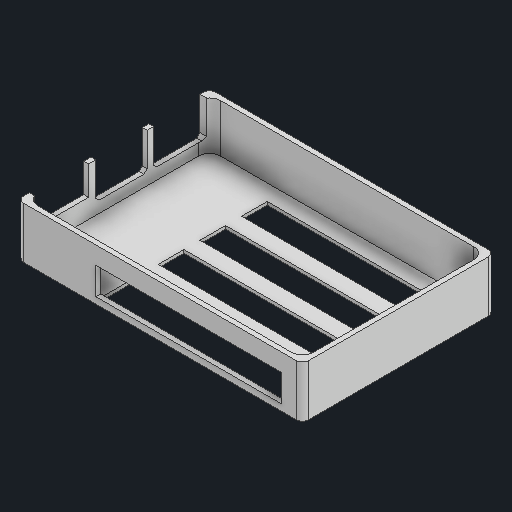
# Autodesk Inventor part: raspi_cover
Saved by Autodesk Inventor 2025 (Build 290162010, 162A)
## iProperties
Created: 2024-09-11
Part Number: raspi_cover
Material: Generic
Document SubType Name: Modeling
Designer: mihir
Density: 1 g/cm^3
Appearance: Default
Author: mihir
Autodesk Inventor part; units mm, degrees
ref_plane "YZ Plane" through (0, 0, 0) normal (1, 0, 0) x (0, 1, 0)
ref_plane "XZ Plane" through (0, 0, 0) normal (0, 1, 0) x (-1, 0, 0)
ref_plane "XY Plane" through (0, 0, 0) normal (0, 0, 1) x (1, 0, 0)
sketch "Sketch1" plane through (0, 0, 0) normal (0, 1, 0) x (-1, 0, 0)
  line L0 (2, 0) -> (87, 0)
  line L1 (89, -2) -> (89, -58)
  line L2 (87, -60) -> (2, -60)
  line L3 (0, -58) -> (0, -2)
  arc A0 (2, 0) -> (0, -2) centre (2, -2) ccw
  arc A1 (0, -58) -> (2, -60) centre (2, -58) ccw
  arc A2 (87, -60) -> (89, -58) centre (87, -58) ccw
  arc A3 (89, -2) -> (87, 0) centre (87, -2) ccw
  point P0 (0, 0)
  point P1 (89, -60)
  point P2 (0, -60)
  dimension "d0" = 60
  dimension "d1" = 89
  dimension "d2" = 2
  constraints: 8 end point, 8 point on circle, 8 tangent, 6 point on line, 4 centre point, 3 equal radius, 2 parallel, 1 horizontal, 1 perpendicular
  measures "d0" distance of point (0, -60) point (0, 0)
  measures "d1" distance of point (89, -60) point (0, -60)
  measures "d2" radius of A0
extrude "Extrusion1" add sketch "Sketch1" along normal blind 1
sketch "Sketch2" plane through (0, 1, 0) normal (0, 1, 0) x (1, 0, 0)
  line L0 (-87, 0) -> (-2, 0)
  line L1 (0, 2) -> (0, 58)
  line L2 (-2, 60) -> (-87, 60)
  line L3 (-89, 58) -> (-89, 2)
  line L4 (-89, 58) -> (-89, 2) projected
  line L5 (-87, 0) -> (-2, 0) projected
  line L6 (0, 2) -> (0, 58) projected
  line L7 (-2, 60) -> (-87, 60) projected
  arc A0 (-89, 2) -> (-87, 0) centre (-87, 2) ccw
  arc A1 (-87, 60) -> (-89, 58) centre (-87, 58) ccw
  arc A2 (0, 58) -> (-2, 60) centre (-2, 58) ccw
  arc A3 (-2, 0) -> (0, 2) centre (-2, 2) ccw
  line L8 (-84, 1.5) -> (-5, 1.5)
  line L9 (-1.5, 5) -> (-1.5, 55)
  line L10 (-5, 58.5) -> (-84, 58.5)
  line L11 (-87.5, 55) -> (-87.5, 5)
  arc A4 (-5, 1.5) -> (-1.5, 5) centre (-5, 5) ccw
  arc A5 (-1.5, 55) -> (-5, 58.5) centre (-5, 55) ccw
  arc A6 (-84, 58.5) -> (-87.5, 55) centre (-84, 55) ccw
  arc A7 (-87.5, 5) -> (-84, 1.5) centre (-84, 5) ccw
  point P0 (0, 0)
  dimension "d5" = 2
  dimension "d6" = 1.5
  dimension "d7" = 1.5
  dimension "d8" = 1.5
  dimension "d9" = 1.5
  dimension "d10" = 3.5
  constraints: 16 end point, 16 point on circle, 16 tangent, 8 centre point, 6 equal radius, 4 collinear, 4 parallel, 2 horizontal, 2 perpendicular
  measures "d5" radius of A0
  measures "d6" distance between parallel lines of L0 L8
  measures "d7" distance between parallel lines of L2 L10
  measures "d8" distance between parallel lines of L3 L11
  measures "d9" distance between parallel lines of L6 L9
  measures "d10" radius of A4
extrude "Extrusion2" add sketch "Sketch2" along normal blind 15
sketch "Sketch3" plane through (-87, 0, 0) normal (0, 0, 1) x (1, 0, 0)
  line L0 (22.5, 10.5) -> (80.5, 10.5)
  line L1 (80.5, 10.5) -> (80.5, 2)
  line L2 (80.5, 2) -> (22.5, 2)
  line L3 (22.5, 2) -> (22.5, 10.5)
  line L4 (87, 0) -> (87, 16) projected
  line L5 (0, 0) -> (85, 0) projected
  dimension "d13" = 58
  dimension "d14" = 8.5
  dimension "d15" = 6.5
  dimension "d16" = 2
  constraints: 8 end point, 2 parallel, 1 horizontal, 1 perpendicular
  measures "d13" distance of L0.start L0.end
  measures "d14" distance of L0.end L1.end
  measures "d15" distance between parallel lines of L4 L1
  measures "d16" distance between parallel lines of L5 L2
extrude "Extrusion3" cut sketch "Sketch3" against normal up to surface (1.5 mm away)
sketch "Sketch4" plane through (0, 1, 0) normal (0, 1, 0) x (1, 0, 0)
  line L0 (-64.5, 1.5) -> (-6.5, 1.5) projected
  line L1 (-64.5, 2.5) -> (-6.5, 2.5)
  line L2 (-6.5, 2.5) -> (-6.5, 14.5)
  line L3 (-6.5, 14.5) -> (-64.5, 14.5)
  line L4 (-64.5, 14.5) -> (-64.5, 2.5)
  line L5 (-6.5, 1.5) -> (-6.5, 2.5) construction
  point P0 (0, 0)
  dimension "d19" = 12
  dimension "d20" = 58
  dimension "d21" = 1
  constraints: 10 end point, 2 parallel, 1 horizontal, 1 perpendicular, 1 vertical
  measures "d19" distance of L1.end L2.end
  measures "d20" distance of L2.end L3.end
  measures "d21" distance of L0.end L1.end
extrude "Extrusion4" cut sketch "Sketch4" against normal up to surface (1 mm away)
sketch "Sketch5" plane through (0, 1, 0) normal (0, 1, 0) x (1, 0, 0)
  line L0 (-64.5, 19.5) -> (-6.5, 19.5)
  line L1 (-6.5, 19.5) -> (-6.5, 27.5)
  line L2 (-6.5, 27.5) -> (-64.5, 27.5)
  line L3 (-64.5, 27.5) -> (-64.5, 19.5)
  line L4 (-64.5, 2.5) -> (-64.5, 14.5) projected
  line L5 (-64.5, 14.5) -> (-6.5, 14.5) projected
  line L6 (-64.5, 32.5) -> (-6.5, 32.5)
  line L7 (-6.5, 32.5) -> (-6.5, 40.5)
  line L8 (-6.5, 40.5) -> (-64.5, 40.5)
  line L9 (-64.5, 40.5) -> (-64.5, 32.5)
  line L10 (-64.5, 45.5) -> (-6.5, 45.5)
  line L11 (-6.5, 45.5) -> (-6.5, 53.5)
  line L12 (-6.5, 53.5) -> (-64.5, 53.5)
  line L13 (-64.5, 53.5) -> (-64.5, 45.5)
  point P0 (0, 0)
  dimension "d24" = 8
  dimension "d25" = 58
  dimension "d26" = 5
  dimension "d27" = 5
  dimension "d28" = 8
  dimension "d29" = 58
  dimension "d30" = 5
  dimension "d31" = 8
  constraints: 24 end point, 6 parallel, 4 collinear, 3 horizontal, 3 perpendicular
  measures "d24" distance of L2.end L0.start
  measures "d25" distance of L1.end L2.end
  measures "d26" distance between parallel lines of L5 L0
  measures "d27" distance between parallel lines of L2 L6
  measures "d28" distance of L8.end L6.start
  measures "d29" distance of L7.end L8.end
  measures "d30" distance between parallel lines of L8 L10
  measures "d31" distance of L12.end L10.start
extrude "Extrusion5" cut sketch "Sketch5" against normal up to surface (1 mm away)
sketch "Sketch6" plane through (-89, 0, -58) normal (-1, 0, 0) x (0, 0, 1)
  line L0 (54.25, 7) -> (37.25, 7)
  line L1 (37.25, 7) -> (37.25, 16)
  line L2 (37.25, 16) -> (54.25, 16)
  line L3 (54.25, 16) -> (54.25, 7)
  line L4 (0, 0) -> (56, 0) projected
  line L5 (0, 16) -> (56, 16) projected
  line L6 (58, 0) -> (58, 16) projected
  dimension "d34" = 7
  dimension "d35" = 3.75
  dimension "d36" = 17
  constraints: 8 end point, 2 parallel, 1 collinear, 1 horizontal, 1 perpendicular
  measures "d34" distance between parallel lines of L4 L0
  measures "d35" distance between parallel lines of L6 L3
  measures "d36" distance of L0.start L0.end
extrude "Extrusion6" cut sketch "Sketch6" against normal blind 2
sketch "Sketch7" plane through (-89, 0, -58) normal (-1, 0, 0) x (0, 0, 1)
  line L0 (35, 16) -> (19, 16)
  line L1 (19, 16) -> (19, 5.6)
  line L2 (19, 5.6) -> (20, 4.6)
  line L3 (20, 4.6) -> (34, 4.6)
  line L4 (34, 4.6) -> (35, 5.6)
  line L5 (35, 5.6) -> (35, 16)
  line L6 (37.25, 7) -> (37.25, 16) projected
  line L7 (0, 16) -> (37.25, 16) projected
  line L8 (0, 0) -> (56, 0) projected
  line L9 (2, 4.6) -> (16, 4.6)
  line L10 (16, 4.6) -> (17, 5.6)
  line L11 (17, 5.6) -> (17, 16)
  line L12 (17, 16) -> (1, 16)
  line L13 (1, 16) -> (1, 5.6)
  line L14 (1, 5.6) -> (2, 4.6)
  point P0 (58, 0)
  point P1 (17, 16)
  point P2 (1, 16)
  dimension "d39" = 2.25
  dimension "d40" = 14
  dimension "d41" = 16
  dimension "d42" = 4.6
  dimension "d45" = 18
  constraints: 24 end point, 2 collinear, 2 equal length, 2 horizontal, 2 parallel, 2 perpendicular, 11 other
  measures "d39" distance between parallel lines of L6 L5
  measures "d40" distance of L2.end L3.end
  measures "d41" distance of L0.start L0.end
  measures "d42" distance between parallel lines of L8 L3
  measures "d45" distance of L2.end L9.start
extrude "Extrusion7" cut sketch "Sketch7" against normal blind 2.5
body "Solid1"
